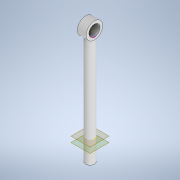
# Autodesk Inventor part: handle with hole
Saved by Autodesk Inventor 2020.4 (Build 244396000, 396)
## iProperties
Created: 2023-07-18
Part Number: handle with hole
Material: Generic
Document SubType Name: Modeling
Designer: Paul
Density: 1 g/cm^3
Appearance: Default
Author: Paul
Autodesk Inventor part; units mm, degrees
ref_plane "YZ Plane" through (0, 0, 0) normal (1, 0, 0) x (0, 1, 0)
ref_plane "XZ Plane" through (0, 0, 0) normal (0, 1, 0) x (-1, 0, 0)
ref_plane "XY Plane" through (0, 0, 0) normal (0, 0, 1) x (1, 0, 0)
ref_plane "Work Plane2" through (-6.35, 0, 0) normal (-1, 0, 0) x (0, 0, 1)
ref_plane "Work Plane3" through (0, 0, 0) normal (1, 0, 0) x (0, 0, -1)
sketch "Sketch3" plane through (0, 0, 0) normal (1, 0, 0) x (0, 0, -1)
  circle A0 centre (0, 0) radius 5.08
  dimension "d35" = 10.16
  constraints: 1 centre point, 1 coincident
  measures "d35" diameter of A0
extrude "Extrusion2" add sketch "Sketch3" along normal blind 101.6 and the other way blind 25.4
sketch "Sketch5" plane through (101.6, 0, 0) normal (1, 0, 0) x (0, 0, -1)
  circle A0 centre (0, 0) radius 5.08 projected
ref_plane "Work Plane1" through (-6.35, 0, 18.2681) normal (0, 1, 0) x (1, 0, 0)
sketch "Sketch6" plane through (-6.35, 0, 18.2681) normal (0, 1, 0) x (1, 0, 0)
  point P0 (6.35, 18.2681)
sketch "Sketch7" plane through (-6.35, 0, 18.2681) normal (0, 1, 0) x (1, 0, 0)
  line L0 (107.95, 13.1881) -> (107.95, 23.3481) projected
  line L1 (107.95, 18.2681) -> (114.3, 18.2681)
  circle A0 centre (114.3, 18.2681) radius 6.35
  circle A1 centre (114.3, 18.2681) radius 9.525
  point P0 (6.35, 18.2681)
  dimension "d50" = 6.35
  dimension "d51" = 19.05
  constraints: 2 coincident, 2 end point, 1 centre point, 1 horizontal, 1 horizontal alignment, 1 midpoint, 2 other
  measures "d50" distance of L1.start L1.end
  measures "d51" diameter of A1
extrude "Extrusion4" add sketch "Sketch7" along normal mid plane 10.16
sketch "Sketch8" plane through (107.95, 5.08, 0) normal (0, 1, 0) x (1, 0, 0)
  point P0 (-107.95, 0)
equation "\"HR\" = 7.874"
equation "\"PR\" = 5.588"
equation "\"HA\" = 55deg"
body "Solid1"
